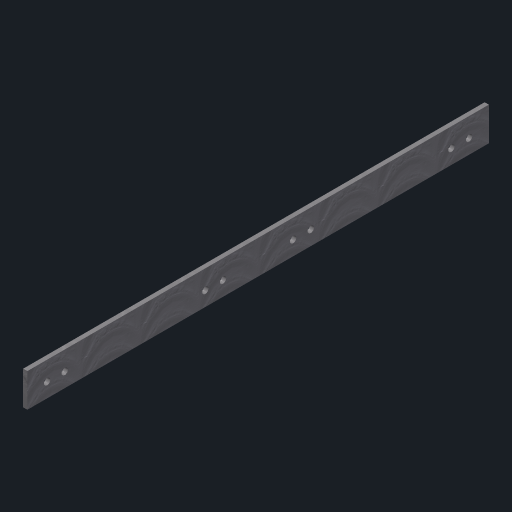
# Autodesk Inventor part: PLENTINA_CANALETA_MOVIL
Saved by Autodesk Inventor 2024.3 (Build 283343000, 343)
## iProperties
Created: 2024-07-24
Part Number: PLENTINA_CANALETA_MOVIL
Material: Steel, Mild, Welded
Document SubType Name: Modeling
Designer: Niler
Density: 7.85 g/cm^3
Appearance: Weld - Steel Mild
Author: Niler
Autodesk Inventor part; units mm, degrees
ref_plane "YZ Plane" through (0, 0, 0) normal (1, 0, 0) x (0, 1, 0)
ref_plane "XZ Plane" through (0, 0, 0) normal (0, 1, 0) x (-1, 0, 0)
ref_plane "XY Plane" through (0, 0, 0) normal (0, 0, 1) x (1, 0, 0)
sketch "Sketch1" plane through (0, 0, 0) normal (1, 0, 0) x (0, 1, 0)
  line L0 (-12.7, 175) -> (12.7, 175)
  line L1 (12.7, 175) -> (12.7, -175)
  line L2 (12.7, -175) -> (-12.7, -175)
  line L3 (-12.7, -175) -> (-12.7, 175)
  line L4 (-12.7, 175) -> (12.7, -175) construction
  line L5 (12.7, 175) -> (-12.7, -175) construction
  point P0 (0, 0)
  dimension "d0" = 25.4
  dimension "d1" = 350
  constraints: 12 end point, 2 midpoint, 2 parallel, 1 horizontal, 1 perpendicular
  measures "d0" distance of L1.end L2.end
  measures "d1" distance of L0.end L1.end
extrude "Extrusion1" add sketch "Sketch1" along normal blind 3.175
sketch "Sketch2" plane through (3.175, 0, 0) normal (1, 0, 0) x (0, 0, -1)
  line L0 (175, -12.7) -> (175, 12.7) projected
  line L1 (175, 12.7) -> (-175, 12.7) projected
  line L2 (-175, 12.7) -> (-175, -12.7) projected
  line L3 (-175, -12.7) -> (175, -12.7) projected
  circle A0 centre (-160, -1.68) radius 2.5
  line L4 (175, 12.7) -> (-175, 12.7) projected
  line L5 (0, 12.7) -> (0, -12.7)
  circle A1 centre (160, -1.68) radius 2.5
  circle A2 centre (-146.6, -1.68) radius 2.5
  circle A3 centre (146.6, -1.68) radius 2.5
  point P0 (0, 0)
  dimension "d4" = 5
  dimension "d5" = 14.38
  dimension "d6" = 15
  dimension "d9" = 13.4
  constraints: 4 centre point, 2 end point, 2 midpoint, 2 symmetric about line, 1 equal radius, 1 horizontal alignment, 2 other
  measures "d4" diameter of A0
  measures "d5" distance from line of A0.centre L1
  measures "d6" distance from line of L2 A0.centre
  measures "d9" distance of A0.centre A2.centre
extrude "Extrusion2" cut sketch "Sketch2" against normal through all contours A0 | A1 | A2 | A3
sketch "Sketch3" plane through (3.175, 0, 0) normal (1, 0, 0) x (0, 0, -1)
  circle A0 centre (-160, -1.68) radius 2.5 projected
  circle A1 centre (146.6, -1.68) radius 2.5 projected
  circle A2 centre (160, -1.68) radius 2.5 projected
  circle A3 centre (-146.6, -1.68) radius 2.5 projected
  line L0 (175, -12.7) -> (175, 12.7) projected
  line L1 (175, 12.7) -> (-175, 12.7) projected
  line L2 (-175, 12.7) -> (-175, -12.7) projected
  line L3 (-175, -12.7) -> (175, -12.7) projected
  circle A4 centre (-160, -1.68) radius 2.5
  circle A5 centre (-146.6, -1.68) radius 2.5
  circle A6 centre (-40, -1.68) radius 2.5
  circle A7 centre (-26.6, -1.68) radius 2.5
  line L4 (0, 0) -> (0, 12.7)
  circle A8 centre (40, -1.68) radius 2.5
  circle A9 centre (26.6, -1.68) radius 2.5
  dimension "d12" = 120
  constraints: 6 centre point, 2 coincident, 2 concentric, 2 end point, 2 symmetric about line, 1 horizontal, 1 midpoint, 6 other
  measures "d12" distance of A4.centre A6.centre
extrude "Extrusion3" cut sketch "Sketch3" against normal through all contours A6 | A7 | A8 | A9
body "Solid1"
